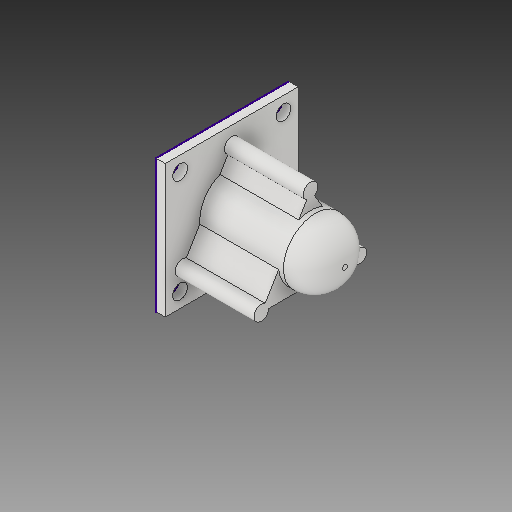
# Autodesk Inventor part: キャスター
Saved by Autodesk Inventor 2018.2 (Build 222227000, 227)
## iProperties
Created: 2019-04-22
Part Number: キャスター
Material: PAEK 樹脂
Document SubType Name: Modeling
Designer: Eiji Nishizawa
Density: 1.32 g/cm^3
Appearance: 滑らか - 白
Author: Eiji Nishizawa
Autodesk Inventor part; units mm, degrees
ref_plane "YZ Plane" through (0, 0, 0) normal (1, 0, 0) x (0, 1, 0)
ref_plane "XZ Plane" through (0, 0, 0) normal (0, 1, 0) x (-1, 0, 0)
ref_plane "XY Plane" through (0, 0, 0) normal (0, 0, 1) x (1, 0, 0)
sketch "スケッチ1" plane through (0, 0, 0) normal (1, 0, 0) x (0, 1, 0)
  line L0 (13.5, 13.5) -> (-13.5, 13.5)
  line L1 (-13.5, 13.5) -> (-13.5, -13.5)
  line L2 (-13.5, -13.5) -> (13.5, -13.5)
  line L3 (13.5, -13.5) -> (13.5, 13.5)
  circle A0 centre (0, 0) radius 6.5
  circle A1 centre (10.5, 10.5) radius 1.5
  circle A2 centre (10.5, -10.5) radius 1.5
  circle A3 centre (-10.5, -10.5) radius 1.5
  circle A4 centre (-10.5, 10.5) radius 1.5
  dimension "d0" = 27
  dimension "d1" = 27
  dimension "d2" = 13.5
  dimension "d3" = 13.5
  dimension "d4" = 13.5
  dimension "d5" = 13.5
  dimension "d6" = 13
  dimension "d7" = 3
  dimension "d8" = 3
  dimension "d9" = 3
  dimension "d10" = 3
  dimension "d11" = 3
  dimension "d12" = 3
  dimension "d13" = 3
  dimension "d14" = 3
  dimension "d15" = 3
  dimension "d16" = 3
  dimension "d17" = 3
  dimension "d18" = 3
  constraints: 8 end point, 5 centre point, 2 parallel, 1 coincident, 1 horizontal, 1 perpendicular
  measures "d0" distance between parallel lines of L1 L3
  measures "d1" distance between parallel lines of L2 L0
  measures "d2" distance from line of point (0, 0) L0
  measures "d3" distance from line of point (0, 0) L2
  measures "d4" distance from line of point (0, 0) L1
  measures "d5" distance from line of L3 point (0, 0)
  measures "d6" diameter of A0
  measures "d7" distance from line of L0 A1.centre
  measures "d8" distance from line of L3 A1.centre
  measures "d9" diameter of A1
  measures "d10" distance from line of L2 A2.centre
  measures "d11" distance from line of L3 A2.centre
  measures "d12" diameter of A2
  measures "d13" distance from line of L0 A4.centre
  measures "d14" distance from line of L1 A4.centre
  measures "d15" diameter of A4
  measures "d16" distance from line of L1 A3.centre
  measures "d17" distance from line of L2 A3.centre
  measures "d18" diameter of A3
extrude "押し出し1" add sketch "スケッチ1" along normal blind 2
extrude "押し出し2" add sketch "スケッチ1" along normal blind 25 contours A0
fillet "フィレット1" radius 6 1 edges at (25, -6.5, 0)
sketch "スケッチ2" plane through (2, 0, 0) normal (1, 0, 0) x (0, 0, -1)
  circle A0 centre (0, 10) radius 1.5
  circle A1 centre (-10, -6.5) radius 1.5
  circle A2 centre (10, -6.5) radius 1.3994
  line L0 (0, 10) -> (10, -6.5)
  line L1 (10, -6.5) -> (-10, -6.5)
  line L2 (0, 10) -> (-10, -6.5)
  line L3 (13.5, 13.5) -> (-13.5, 13.5) projected
  line L4 (13.5, -13.5) -> (13.5, 13.5) projected
  line L5 (-13.5, 13.5) -> (-13.5, -13.5) projected
  line L6 (-13.5, -13.5) -> (13.5, -13.5) projected
  point P0 (0, 0)
  dimension "d25" = 3.5
  dimension "d26" = 3.5
  dimension "d27" = 3.5
  dimension "d28" = 2.7988
  dimension "d29" = 7
  dimension "d30" = 3
  dimension "d31" = 3
  constraints: 6 end point, 3 centre point, 1 horizontal
  measures "d25" distance from line of L3 L0.start
  measures "d26" distance from line of L4 L0.end
  measures "d27" distance from line of L5 L1.end
  measures "d28" diameter of A2
  measures "d29" distance from line of L6 L0.end
  measures "d30" diameter of A0
  measures "d31" diameter of A1
extrude "押し出し3" add sketch "スケッチ2" along normal blind 16 contours A0 L0 L2 | L2 L0 A0 | A0 L0 A2 L1 A1 L2 | L2 L1 A1 | A1 L1 L2 | L0 L1 A2 | A2 L1 L0
